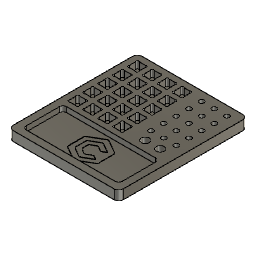
Bamboo Tray (Fusion) (Autodesk Fusion 360 design; units mm, degrees)
Autodesk Fusion 360 part; units mm, degrees
sketch "Sketch1" plane through (0, 0, 0) normal (0, 0, 1) x (1, 0, 0)
  line L0 (0, 0) -> (148, 0)
  line L1 (148, 0) -> (148, 173)
  line L2 (148, 173) -> (0, 173)
  line L3 (0, 173) -> (0, 0)
  dimension "d1" = 148
  dimension "d2" = 173
  constraint horizontal L0
  constraint vertical L1
  constraint horizontal L2
  constraint vertical L3
  constraint coincident L0.start L3.end
  measures "d1" distance of L0.start L0.end
  measures "d2" distance of L0.start L2.end
extrude "Extrude1" add sketch "Sketch1" along normal blind 12.7
sketch "Sketch2" plane through (0, 0, 12.7) normal (0, 0, 1) x (-1, 0, 0)
  line L0 (0, -173) -> (0, 0) construction
  line L1 (0, 0) -> (-148, 0) construction
  line L2 (-148, 0) -> (-148, -173) construction
  line L3 (-11.2739, -71.314) -> (-18.7691, -71.314)
  line L4 (-21.5019, -74.0964) -> (-21.5019, -81.9465)
  line L5 (-18.7712, -84.7264) -> (-11.1924, -84.7264)
  line L6 (-8.4537, -81.9513) -> (-8.4537, -74.0071)
  line L7 (-8.5338, -71.2781) -> (-21.432, -84.6864) construction
  line L8 (-21.4944, -71.3042) -> (-8.4323, -84.7713) construction
  arc A0 (-11.1924, -84.7264) -> (-8.4537, -81.9513) centre (-9.79, -83.3716) ccw
  arc A1 (-21.5019, -81.9465) -> (-18.7712, -84.7264) centre (-20.0802, -83.2811) ccw
  arc A2 (-8.4537, -74.0071) -> (-11.2739, -71.314) centre (-9.8857, -72.6834) ccw
  arc A3 (-18.7691, -71.314) -> (-21.5019, -74.0964) centre (-20.1368, -72.704) ccw
  line L9 (-28.4537, -81.9513) -> (-28.4537, -74.0071)
  arc A4 (-28.4537, -74.0071) -> (-31.2739, -71.314) centre (-29.8857, -72.6834) ccw
  line L10 (-31.2739, -71.314) -> (-38.7691, -71.314)
  arc A5 (-38.7691, -71.314) -> (-41.5019, -74.0964) centre (-40.1368, -72.704) ccw
  line L11 (-41.5019, -74.0964) -> (-41.5019, -81.9465)
  arc A6 (-41.5019, -81.9465) -> (-38.7712, -84.7264) centre (-40.0802, -83.2811) ccw
  line L12 (-38.7712, -84.7264) -> (-31.1924, -84.7264)
  arc A7 (-31.1924, -84.7264) -> (-28.4537, -81.9513) centre (-29.79, -83.3716) ccw
  line L13 (-48.4537, -81.9513) -> (-48.4537, -74.0071)
  arc A8 (-48.4537, -74.0071) -> (-51.2739, -71.314) centre (-49.8857, -72.6834) ccw
  line L14 (-51.2739, -71.314) -> (-58.7691, -71.314)
  arc A9 (-58.7691, -71.314) -> (-61.5019, -74.0964) centre (-60.1368, -72.704) ccw
  line L15 (-61.5019, -74.0964) -> (-61.5019, -81.9465)
  arc A10 (-61.5019, -81.9465) -> (-58.7712, -84.7264) centre (-60.0802, -83.2811) ccw
  line L16 (-58.7712, -84.7264) -> (-51.1924, -84.7264)
  arc A11 (-51.1924, -84.7264) -> (-48.4537, -81.9513) centre (-49.79, -83.3716) ccw
  line L17 (-68.4537, -81.9513) -> (-68.4537, -74.0071)
  arc A12 (-68.4537, -74.0071) -> (-71.2739, -71.314) centre (-69.8857, -72.6834) ccw
  line L18 (-71.2739, -71.314) -> (-78.7691, -71.314)
  arc A13 (-78.7691, -71.314) -> (-81.5019, -74.0964) centre (-80.1368, -72.704) ccw
  line L19 (-81.5019, -74.0964) -> (-81.5019, -81.9465)
  arc A14 (-81.5019, -81.9465) -> (-78.7712, -84.7264) centre (-80.0802, -83.2811) ccw
  line L20 (-78.7712, -84.7264) -> (-71.1924, -84.7264)
  arc A15 (-71.1924, -84.7264) -> (-68.4537, -81.9513) centre (-69.79, -83.3716) ccw
  line L21 (-8.4537, -101.9513) -> (-8.4537, -94.0071)
  arc A16 (-8.4537, -94.0071) -> (-11.2739, -91.314) centre (-9.8857, -92.6834) ccw
  line L22 (-11.2739, -91.314) -> (-18.7691, -91.314)
  arc A17 (-18.7691, -91.314) -> (-21.5019, -94.0964) centre (-20.1368, -92.704) ccw
  line L23 (-21.5019, -94.0964) -> (-21.5019, -101.9465)
  arc A18 (-21.5019, -101.9465) -> (-18.7712, -104.7264) centre (-20.0802, -103.2811) ccw
  line L24 (-18.7712, -104.7264) -> (-11.1924, -104.7264)
  arc A19 (-11.1924, -104.7264) -> (-8.4537, -101.9513) centre (-9.79, -103.3716) ccw
  line L25 (-28.4537, -101.9513) -> (-28.4537, -94.0071)
  arc A20 (-28.4537, -94.0071) -> (-31.2739, -91.314) centre (-29.8857, -92.6834) ccw
  line L26 (-31.2739, -91.314) -> (-38.7691, -91.314)
  arc A21 (-38.7691, -91.314) -> (-41.5019, -94.0964) centre (-40.1368, -92.704) ccw
  line L27 (-41.5019, -94.0964) -> (-41.5019, -101.9465)
  arc A22 (-41.5019, -101.9465) -> (-38.7712, -104.7264) centre (-40.0802, -103.2811) ccw
  line L28 (-38.7712, -104.7264) -> (-31.1924, -104.7264)
  arc A23 (-31.1924, -104.7264) -> (-28.4537, -101.9513) centre (-29.79, -103.3716) ccw
  line L29 (-48.4537, -101.9513) -> (-48.4537, -94.0071)
  arc A24 (-48.4537, -94.0071) -> (-51.2739, -91.314) centre (-49.8857, -92.6834) ccw
  line L30 (-51.2739, -91.314) -> (-58.7691, -91.314)
  arc A25 (-58.7691, -91.314) -> (-61.5019, -94.0964) centre (-60.1368, -92.704) ccw
  line L31 (-61.5019, -94.0964) -> (-61.5019, -101.9465)
  arc A26 (-61.5019, -101.9465) -> (-58.7712, -104.7264) centre (-60.0802, -103.2811) ccw
  line L32 (-58.7712, -104.7264) -> (-51.1924, -104.7264)
  arc A27 (-51.1924, -104.7264) -> (-48.4537, -101.9513) centre (-49.79, -103.3716) ccw
  line L33 (-68.4537, -101.9513) -> (-68.4537, -94.0071)
  arc A28 (-68.4537, -94.0071) -> (-71.2739, -91.314) centre (-69.8857, -92.6834) ccw
  line L34 (-71.2739, -91.314) -> (-78.7691, -91.314)
  arc A29 (-78.7691, -91.314) -> (-81.5019, -94.0964) centre (-80.1368, -92.704) ccw
  line L35 (-81.5019, -94.0964) -> (-81.5019, -101.9465)
  arc A30 (-81.5019, -101.9465) -> (-78.7712, -104.7264) centre (-80.0802, -103.2811) ccw
  line L36 (-78.7712, -104.7264) -> (-71.1924, -104.7264)
  arc A31 (-71.1924, -104.7264) -> (-68.4537, -101.9513) centre (-69.79, -103.3716) ccw
  line L37 (-8.4537, -121.9513) -> (-8.4537, -114.0071)
  arc A32 (-8.4537, -114.0071) -> (-11.2739, -111.314) centre (-9.8857, -112.6834) ccw
  line L38 (-11.2739, -111.314) -> (-18.7691, -111.314)
  arc A33 (-18.7691, -111.314) -> (-21.5019, -114.0964) centre (-20.1368, -112.704) ccw
  line L39 (-21.5019, -114.0964) -> (-21.5019, -121.9465)
  arc A34 (-21.5019, -121.9465) -> (-18.7712, -124.7264) centre (-20.0802, -123.2811) ccw
  line L40 (-18.7712, -124.7264) -> (-11.1924, -124.7264)
  arc A35 (-11.1924, -124.7264) -> (-8.4537, -121.9513) centre (-9.79, -123.3716) ccw
  line L41 (-28.4537, -121.9513) -> (-28.4537, -114.0071)
  arc A36 (-28.4537, -114.0071) -> (-31.2739, -111.314) centre (-29.8857, -112.6834) ccw
  line L42 (-31.2739, -111.314) -> (-38.7691, -111.314)
  arc A37 (-38.7691, -111.314) -> (-41.5019, -114.0964) centre (-40.1368, -112.704) ccw
  line L43 (-41.5019, -114.0964) -> (-41.5019, -121.9465)
  arc A38 (-41.5019, -121.9465) -> (-38.7712, -124.7264) centre (-40.0802, -123.2811) ccw
  line L44 (-38.7712, -124.7264) -> (-31.1924, -124.7264)
  arc A39 (-31.1924, -124.7264) -> (-28.4537, -121.9513) centre (-29.79, -123.3716) ccw
  line L45 (-48.4537, -121.9513) -> (-48.4537, -114.0071)
  arc A40 (-48.4537, -114.0071) -> (-51.2739, -111.314) centre (-49.8857, -112.6834) ccw
  line L46 (-51.2739, -111.314) -> (-58.7691, -111.314)
  arc A41 (-58.7691, -111.314) -> (-61.5019, -114.0964) centre (-60.1368, -112.704) ccw
  line L47 (-61.5019, -114.0964) -> (-61.5019, -121.9465)
  arc A42 (-61.5019, -121.9465) -> (-58.7712, -124.7264) centre (-60.0802, -123.2811) ccw
  line L48 (-58.7712, -124.7264) -> (-51.1924, -124.7264)
  arc A43 (-51.1924, -124.7264) -> (-48.4537, -121.9513) centre (-49.79, -123.3716) ccw
  line L49 (-68.4537, -121.9513) -> (-68.4537, -114.0071)
  arc A44 (-68.4537, -114.0071) -> (-71.2739, -111.314) centre (-69.8857, -112.6834) ccw
  line L50 (-71.2739, -111.314) -> (-78.7691, -111.314)
  arc A45 (-78.7691, -111.314) -> (-81.5019, -114.0964) centre (-80.1368, -112.704) ccw
  line L51 (-81.5019, -114.0964) -> (-81.5019, -121.9465)
  arc A46 (-81.5019, -121.9465) -> (-78.7712, -124.7264) centre (-80.0802, -123.2811) ccw
  line L52 (-78.7712, -124.7264) -> (-71.1924, -124.7264)
  arc A47 (-71.1924, -124.7264) -> (-68.4537, -121.9513) centre (-69.79, -123.3716) ccw
  line L53 (-8.4537, -141.9513) -> (-8.4537, -134.0071)
  arc A48 (-8.4537, -134.0071) -> (-11.2739, -131.314) centre (-9.8857, -132.6834) ccw
  line L54 (-11.2739, -131.314) -> (-18.7691, -131.314)
  arc A49 (-18.7691, -131.314) -> (-21.5019, -134.0964) centre (-20.1368, -132.704) ccw
  line L55 (-21.5019, -134.0964) -> (-21.5019, -141.9465)
  arc A50 (-21.5019, -141.9465) -> (-18.7712, -144.7264) centre (-20.0802, -143.2811) ccw
  line L56 (-18.7712, -144.7264) -> (-11.1924, -144.7264)
  arc A51 (-11.1924, -144.7264) -> (-8.4537, -141.9513) centre (-9.79, -143.3716) ccw
  line L57 (-28.4537, -141.9513) -> (-28.4537, -134.0071)
  arc A52 (-28.4537, -134.0071) -> (-31.2739, -131.314) centre (-29.8857, -132.6834) ccw
  line L58 (-31.2739, -131.314) -> (-38.7691, -131.314)
  arc A53 (-38.7691, -131.314) -> (-41.5019, -134.0964) centre (-40.1368, -132.704) ccw
  line L59 (-41.5019, -134.0964) -> (-41.5019, -141.9465)
  arc A54 (-41.5019, -141.9465) -> (-38.7712, -144.7264) centre (-40.0802, -143.2811) ccw
  line L60 (-38.7712, -144.7264) -> (-31.1924, -144.7264)
  arc A55 (-31.1924, -144.7264) -> (-28.4537, -141.9513) centre (-29.79, -143.3716) ccw
  line L61 (-48.4537, -141.9513) -> (-48.4537, -134.0071)
  arc A56 (-48.4537, -134.0071) -> (-51.2739, -131.314) centre (-49.8857, -132.6834) ccw
  line L62 (-51.2739, -131.314) -> (-58.7691, -131.314)
  arc A57 (-58.7691, -131.314) -> (-61.5019, -134.0964) centre (-60.1368, -132.704) ccw
  line L63 (-61.5019, -134.0964) -> (-61.5019, -141.9465)
  arc A58 (-61.5019, -141.9465) -> (-58.7712, -144.7264) centre (-60.0802, -143.2811) ccw
  line L64 (-58.7712, -144.7264) -> (-51.1924, -144.7264)
  arc A59 (-51.1924, -144.7264) -> (-48.4537, -141.9513) centre (-49.79, -143.3716) ccw
  line L65 (-68.4537, -141.9513) -> (-68.4537, -134.0071)
  arc A60 (-68.4537, -134.0071) -> (-71.2739, -131.314) centre (-69.8857, -132.6834) ccw
  line L66 (-71.2739, -131.314) -> (-78.7691, -131.314)
  arc A61 (-78.7691, -131.314) -> (-81.5019, -134.0964) centre (-80.1368, -132.704) ccw
  line L67 (-81.5019, -134.0964) -> (-81.5019, -141.9465)
  arc A62 (-81.5019, -141.9465) -> (-78.7712, -144.7264) centre (-80.0802, -143.2811) ccw
  line L68 (-78.7712, -144.7264) -> (-71.1924, -144.7264)
  arc A63 (-71.1924, -144.7264) -> (-68.4537, -141.9513) centre (-69.79, -143.3716) ccw
  line L69 (-8.4537, -161.9513) -> (-8.4537, -154.0071)
  arc A64 (-8.4537, -154.0071) -> (-11.2739, -151.314) centre (-9.8857, -152.6834) ccw
  line L70 (-11.2739, -151.314) -> (-18.7691, -151.314)
  arc A65 (-18.7691, -151.314) -> (-21.5019, -154.0964) centre (-20.1368, -152.704) ccw
  line L71 (-21.5019, -154.0964) -> (-21.5019, -161.9465)
  arc A66 (-21.5019, -161.9465) -> (-18.7712, -164.7264) centre (-20.0802, -163.2811) ccw
  line L72 (-18.7712, -164.7264) -> (-11.1924, -164.7264)
  arc A67 (-11.1924, -164.7264) -> (-8.4537, -161.9513) centre (-9.79, -163.3716) ccw
  line L73 (-28.4537, -161.9513) -> (-28.4537, -154.0071)
  arc A68 (-28.4537, -154.0071) -> (-31.2739, -151.314) centre (-29.8857, -152.6834) ccw
  line L74 (-31.2739, -151.314) -> (-38.7691, -151.314)
  arc A69 (-38.7691, -151.314) -> (-41.5019, -154.0964) centre (-40.1368, -152.704) ccw
  line L75 (-41.5019, -154.0964) -> (-41.5019, -161.9465)
  arc A70 (-41.5019, -161.9465) -> (-38.7712, -164.7264) centre (-40.0802, -163.2811) ccw
  line L76 (-38.7712, -164.7264) -> (-31.1924, -164.7264)
  arc A71 (-31.1924, -164.7264) -> (-28.4537, -161.9513) centre (-29.79, -163.3716) ccw
  line L77 (-48.4537, -161.9513) -> (-48.4537, -154.0071)
  arc A72 (-48.4537, -154.0071) -> (-51.2739, -151.314) centre (-49.8857, -152.6834) ccw
  line L78 (-51.2739, -151.314) -> (-58.7691, -151.314)
  arc A73 (-58.7691, -151.314) -> (-61.5019, -154.0964) centre (-60.1368, -152.704) ccw
  line L79 (-61.5019, -154.0964) -> (-61.5019, -161.9465)
  arc A74 (-61.5019, -161.9465) -> (-58.7712, -164.7264) centre (-60.0802, -163.2811) ccw
  line L80 (-58.7712, -164.7264) -> (-51.1924, -164.7264)
  arc A75 (-51.1924, -164.7264) -> (-48.4537, -161.9513) centre (-49.79, -163.3716) ccw
  line L81 (-68.4537, -161.9513) -> (-68.4537, -154.0071)
  arc A76 (-68.4537, -154.0071) -> (-71.2739, -151.314) centre (-69.8857, -152.6834) ccw
  line L82 (-71.2739, -151.314) -> (-78.7691, -151.314)
  arc A77 (-78.7691, -151.314) -> (-81.5019, -154.0964) centre (-80.1368, -152.704) ccw
  line L83 (-81.5019, -154.0964) -> (-81.5019, -161.9465)
  arc A78 (-81.5019, -161.9465) -> (-78.7712, -164.7264) centre (-80.0802, -163.2811) ccw
  line L84 (-78.7712, -164.7264) -> (-71.1924, -164.7264)
  arc A79 (-71.1924, -164.7264) -> (-68.4537, -161.9513) centre (-69.79, -163.3716) ccw
  line L85 (-148, -173) -> (0, -173)
  circle A80 centre (-133, -160.5) radius 3.275
  circle A81 centre (-116, -160.5) radius 3.275
  circle A82 centre (-99, -160.5) radius 3.275
  circle A83 centre (-133, -143.5) radius 3.275
  circle A84 centre (-116, -143.5) radius 3.275
  circle A85 centre (-99, -143.5) radius 3.275
  circle A86 centre (-133, -126.5) radius 3.275
  circle A87 centre (-116, -126.5) radius 3.275
  circle A88 centre (-99, -126.5) radius 3.275
  circle A89 centre (-133, -109.5) radius 3.275
  circle A90 centre (-116, -109.5) radius 3.275
  circle A91 centre (-99, -109.5) radius 3.275
  circle A92 centre (-133, -92.5) radius 3.275
  circle A93 centre (-116, -92.5) radius 3.275
  circle A94 centre (-99, -92.5) radius 3.275
  line L86 (-99, -92.5) -> (-116, -92.5) construction
  circle A95 centre (-106.2904, -77.5) radius 5.375
  circle A96 centre (-126.2904, -77.5) radius 5.375
  line L87 (-138.5, -9.5) -> (-9.5, -9.5)
  line L88 (-9.5, -9.5) -> (-9.5, -63.814)
  line L89 (-9.5, -63.814) -> (-138.5, -63.814)
  line L90 (-138.5, -63.814) -> (-138.5, -9.5)
  line L91 (-138.5, -9.5) -> (-9.5, -63.814) construction
  line L92 (-9.5, -9.5) -> (-138.5, -63.814) construction
  line L93 (-106.2904, -92.5) -> (-106.2904, -77.5) construction
  line L94 (-126.2904, -77.5) -> (-106.2904, -77.5) construction
  point P0 (-15, -78)
  point P1 (-106.2904, -92.5)
  point P2 (-81.5019, -78.0214)
  point P3 (-74, -36.657)
  dimension "d6" = 13
  dimension "d8" = 15
  dimension "d13" = 3.9
  dimension "d14" = 3.9
  dimension "d15" = 3.9
  dimension "d16" = 3.9
  dimension "d19" = -20
  dimension "d20" = -20
  dimension "d27" = 95
  dimension "d28" = 6.55
  dimension "d30" = 30
  dimension "d31" = 50
  dimension "d32" = 17
  dimension "d33" = 17
  dimension "d34" = 15
  dimension "d35" = 12.5
  dimension "d49" = 9.5
  dimension "d50" = 9.5
  dimension "d51" = 9.5
  dimension "d52" = 7.5
  dimension "d56" = 15
  dimension "d61" = 10.75
  dimension "d62" = 20
  dimension "d63" = 9.7096
  constraint perpendicular L3 L4
  constraint parallel L3 L5
  constraint parallel L4 L6
  constraint horizontal L3
  constraint coincident L7 P0
  constraint coincident L8 P0
  constraint coincident L8 A0.centre
  constraint coincident L8.end A0
  constraint coincident L7 A1.centre
  constraint coincident L7.end A1
  constraint coincident L8 A3.centre
  constraint coincident L8.start A3
  constraint coincident L7 A2.centre
  constraint coincident L7.start A2
  constraint coincident A94.centre L86.start
  constraint coincident A93.centre L86.end
  constraint midpoint L19 P2
  constraint horizontal L87
  constraint perpendicular L87 L88
  constraint parallel L87 L89
  constraint parallel L88 L90
  constraint coincident L91 P3
  constraint coincident L92 P3
  constraint coincident P1 L93.start
  constraint coincident A95.centre L93.end
  constraint vertical L93
  constraint equal A95 A96
  constraint coincident A96.centre L94.start
  constraint perpendicular L93 L94
  measures "d6" distance of L7.end L8.end
  measures "d8" distance of L0 P0
  measures "d13" diameter of A0
  measures "d14" diameter of A1
  measures "d15" diameter of A3
  measures "d16" diameter of A2
  measures "d27" distance of P0 L85
  measures "d28" diameter of A80
  measures "d34" distance of L2 A80.centre
  measures "d35" distance of L85 A80.centre
  measures "d49" distance of L1 L87
  measures "d50" distance of L2 L90
  measures "d51" distance of L0 L88
  measures "d52" distance of L3 L89
  measures "d56" distance of P1 A95.centre
  measures "d61" diameter of A96
  measures "d62" distance of A95.centre A96.centre
  measures "d63" distance of A93.centre A95.centre
extrude "Extrude2" cut sketch "Sketch2" against normal blind 9.5 contours L3 L4 L5 L6 A0 A1 A2 A3 | L9 A4 L10 A5 L11 A6 L12 A7 | L13 A8 L14 A9 L15 A10 L16 A11 | L17 A12 L18 A13 L19 A14 L20 A15 | L21 A16 L22 A17 L23 A18 L24 A19 | L25 A20 L26 A21 L27 A22 L28 A23 | L29 A24 L30 A25 L31 A26 L32 A27 | L33 A28 L34 A29 L35 A30 L36 A31 | L37 A32 L38 A33 L39 A34 L40 A35 | L41 A36 L42 A37 L43 A38 L44 A39 | L45 A40 L46 A41 L47 A42 L48 A43 | L49 A44 L50 A45 L51 A46 L52 A47 | L53 A48 L54 A49 L55 A50 L56 A51 | L57 A52 L58 A53 L59 A54 L60 A55 | L61 A56 L62 A57 L63 A58 L64 A59 | L65 A60 L66 A61 L67 A62 L68 A63 | L69 A64 L70 A65 L71 A66 L72 A67 | L73 A68 L74 A69 L75 A70 L76 A71 | L77 A72 L78 A73 L79 A74 L80 A75 | L81 A76 L82 A77 L83 A78 L84 A79 | A80 | A81 | A82 | A83 | A84 | A85 | A86 | A87 | A88 | A89 | A90 | A91 | A92 | A93 | A94
fillet "Fillet1" radius 6 4 edges at (0, 0, 6.35) (148, 0, 6.35) (148, 173, 6.35) (0, 173, 6.35)
ref_plane "WorkPlane1" through (104.5, 75, 7.45) normal (0, 1, 0) x (0, 0, -1)
sketch "Sketch3" plane through (104.5, 75, 7.45) normal (0, 1, 0) x (1, 0, 0)
  line L0 (4.6, -5.25) -> (-4.6, -5.25)
  line L1 (4.6, 5.25) -> (-4.6, 5.25)
  line L2 (4.6, -5.25) -> (-4.6, -5.25)
  line L3 (0, 0) -> (0, -5.25)
  line L4 (4.6, -5.25) -> (3.1243, 5.25) construction
  line L5 (4.6, -5.25) -> (15.1032, -5.25) construction
  line L6 (4.6, 5.25) -> (4.6, 1.25)
  line L7 (4.6, 1.25) -> (3.6865, 1.25)
  line L8 (3.6865, 1.25) -> (3.6865, 5.25)
  line L9 (3.6865, 5.25) -> (4.6, 5.25)
  dimension "d40" = 98
  dimension "d41" = 4
  constraint coincident L3.start origin
  constraint midpoint L0 L3.end
  constraint horizontal L5
  constraint coincident L0.start L2.start
  constraint coincident L1 L4.end
  constraint coincident L1.start L6.start
  constraint perpendicular L1 L6
  constraint coincident L4 L7.end
  constraint perpendicular L6 L7
  constraint coincident L1 L8.end
  constraint perpendicular L1 L8
  measures "d40" angle of L4 L5
  measures "d41" distance of L1.start L6.end
revolve "Revolve1" [suppressed]
extrude "Extrude3" cut sketch "Sketch2" against normal blind 10.5 draft -8 contours A95 | A96
extrude "Extrude4" cut sketch "Sketch2" against normal blind 7 contours L87 L88 L89 L90
fillet "Fillet2" radius 5 4 edges at (9.5, 63.814, 9.2) (9.5, 9.5, 9.2) (138.5, 63.814, 9.2) (138.5, 9.5, 9.2)
sketch "Sketch4" plane through (0, 0, 5.7) normal (0, 0, 1) x (-1, 0, 0)
  arc A0 (-133.5, -9.5) -> (-138.5, -14.5) centre (-133.5, -14.5) ccw
  line L0 (-138.5, -14.5) -> (-138.5, -58.814)
  arc A1 (-138.5, -58.814) -> (-133.5, -63.814) centre (-133.5, -58.814) ccw
  line L1 (-133.5, -63.814) -> (-14.5, -63.814)
  arc A2 (-14.5, -63.814) -> (-9.5, -58.814) centre (-14.5, -58.814) ccw
  line L2 (-9.5, -58.814) -> (-9.5, -14.5)
  arc A3 (-9.5, -14.5) -> (-14.5, -9.5) centre (-14.5, -14.5) ccw
  line L3 (-14.5, -9.5) -> (-133.5, -9.5)
  line L4 (-75.1019, -28.3976) -> (-80.9582, -31.7787)
  arc A4 (-72.8981, -28.3976) -> (-75.1019, -28.3976) centre (-74, -30.3062) ccw
  arc A5 (-65.9399, -33.6873) -> (-67.0418, -31.7787) centre (-68.1438, -33.6873) ccw
  line L5 (-65.9399, -40.4495) -> (-65.9399, -33.6873)
  line L6 (-72.8981, -45.7392) -> (-67.0418, -42.3581)
  arc A6 (-67.0418, -42.3581) -> (-65.9399, -40.4495) centre (-68.1438, -40.4495) ccw
  line L7 (-67.0418, -31.7787) -> (-72.8981, -28.3976)
  arc A7 (-60.0441, -43.8607) -> (-61.0054, -45.6809) centre (-62.248, -43.8607) cw
  line L8 (-60.0441, -30.2834) -> (-60.0441, -43.8607)
  arc A8 (-61.146, -28.3747) -> (-60.0441, -30.2834) centre (-62.248, -30.2834) cw
  arc A9 (-72.8981, -52.5471) -> (-75.1019, -52.5471) centre (-74, -50.6385) cw
  line L9 (-87.1295, -44.6487) -> (-83.1621, -42.3581)
  line L10 (-75.1019, -52.5471) -> (-87.1295, -45.603)
  arc A10 (-87.1295, -29.4881) -> (-87.1295, -28.5338) centre (-86.854, -29.0109) cw
  arc A11 (-75.1019, -21.5897) -> (-72.8981, -21.5897) centre (-74, -23.4983) cw
  line L11 (-72.8981, -21.5897) -> (-61.146, -28.3747)
  line L12 (-87.1295, -28.5338) -> (-75.1019, -21.5897)
  arc A12 (-83.1621, -42.3581) -> (-80.9582, -42.3581) centre (-82.0601, -44.2667) cw
  arc A13 (-87.1295, -45.603) -> (-87.1295, -44.6487) centre (-86.854, -45.1259) cw
  line L13 (-61.0054, -45.6809) -> (-72.8981, -52.5471)
  line L14 (-80.9582, -42.3581) -> (-75.1019, -45.7392)
  arc A14 (-75.1019, -45.7392) -> (-72.8981, -45.7392) centre (-74, -43.8306) ccw
  line L15 (-83.1621, -31.7787) -> (-87.1295, -29.4881)
  arc A15 (-80.9582, -31.7787) -> (-83.1621, -31.7787) centre (-82.0601, -29.87) cw
  line L16 (-74, -63.814) -> (-74, -9.5) construction
  arc A16 (-94.2793, -26.6328) -> (-93.1774, -24.7242) centre (-92.0754, -26.6328) cw
  arc A17 (-54.8229, -24.7238) -> (-53.7209, -26.6324) centre (-55.9248, -26.6324) cw
  line L17 (-93.1774, -24.7242) -> (-75.1022, -14.2882)
  arc A18 (-53.7207, -47.504) -> (-54.8226, -49.4126) centre (-55.9246, -47.504) cw
  line L18 (-53.7209, -26.6324) -> (-53.7207, -47.504)
  line L19 (-54.8226, -49.4126) -> (-72.8978, -59.8486)
  line L20 (-94.2791, -47.5044) -> (-94.2793, -26.6328)
  arc A19 (-93.1771, -49.413) -> (-94.2791, -47.5044) centre (-92.0752, -47.5044) cw
  arc A20 (-75.1022, -14.2882) -> (-72.8983, -14.2882) centre (-74.0002, -16.1968) cw
  arc A21 (-72.8978, -59.8486) -> (-75.1017, -59.8486) centre (-73.9998, -57.94) cw
  line L21 (-75.1017, -59.8486) -> (-93.1771, -49.413)
  line L22 (-72.8983, -14.2882) -> (-54.8229, -24.7238)
  point P0 (-74, -36.657)
  constraint midpoint L1 L16.start
  constraint midpoint L3 L16.end
  constraint midpoint L16 P0
sketch "Sketch5" plane through (0, 0, 4.7) normal (0, 0, 1) x (-1, 0, 0)
  arc A0 (-133, -10) -> (-138, -15) centre (-133, -15) ccw
  line L0 (-138, -15) -> (-138, -58.814)
  arc A1 (-138, -58.814) -> (-133, -63.814) centre (-133, -58.814) ccw
  line L1 (-133, -63.814) -> (-15, -63.814)
  arc A2 (-15, -63.814) -> (-10, -58.814) centre (-15, -58.814) ccw
  line L2 (-10, -58.814) -> (-10, -15)
  arc A3 (-10, -15) -> (-15, -10) centre (-15, -15) ccw
  line L3 (-15, -10) -> (-133, -10)
  line L4 (-74, -63.814) -> (-74, -10) construction
  line L5 (-138, -36.907) -> (-10, -36.907) construction
  line L6 (-44.0656, -28.0911) -> (-44.0656, -45.4544)
  line L7 (-44.0656, -45.4544) -> (-42.6997, -45.4544)
  line L8 (-42.6997, -45.4544) -> (-42.7229, -32.6519)
  line L9 (-42.7229, -32.6519) -> (-42.7692, -30.7998)
  line L10 (-42.7692, -30.7998) -> (-42.7229, -30.7766)
  line L11 (-42.7229, -30.7766) -> (-41.7042, -32.3509)
  line L12 (-41.7042, -32.3509) -> (-33.0226, -45.4544)
  line L13 (-33.0226, -45.4544) -> (-31.5178, -45.4544)
  line L14 (-31.5178, -45.4544) -> (-31.5178, -28.0911)
  line L15 (-31.5178, -28.0911) -> (-32.9069, -28.0911)
  line L16 (-32.9069, -28.0911) -> (-32.9069, -41.1946)
  line L17 (-32.9069, -41.1946) -> (-32.8837, -43.0698)
  line L18 (-32.8837, -43.0698) -> (-32.93, -43.093)
  line L19 (-32.93, -43.093) -> (-33.9486, -41.5187)
  line L20 (-33.9486, -41.5187) -> (-42.9312, -28.0911)
  line L21 (-42.9312, -28.0911) -> (-44.0656, -28.0911)
  spline S0 degree 3 poles (-62.1003, -36.7728) (-62.1003, -43.2087) (-60.2251, -45.7322) (-55.1781, -45.7322) knots 0 0 0 0 1 1 1 1
  spline S1 degree 3 poles (-55.1781, -45.7322) (-50.1544, -45.7322) (-48.256, -43.2087) (-48.256, -36.7728) knots 0 0 0 0 1 1 1 1
  spline S2 degree 3 poles (-48.256, -36.7728) (-48.256, -30.3368) (-50.1775, -27.767) (-55.1781, -27.767) knots 0 0 0 0 1 1 1 1
  spline S3 degree 3 poles (-55.1781, -27.767) (-60.2251, -27.767) (-62.1003, -30.3136) (-62.1003, -36.7728) knots 0 0 0 0 1 1 1 1
  spline S4 degree 3 poles (-60.526, -36.7728) (-60.526, -30.9387) (-59.0212, -29.2487) (-55.2013, -29.2487) knots 0 0 0 0 1 1 1 1
  spline S5 degree 3 poles (-55.2013, -29.2487) (-51.3582, -29.2487) (-49.8302, -30.9387) (-49.8302, -36.7728) knots 0 0 0 0 1 1 1 1
  spline S6 degree 3 poles (-49.8302, -36.7728) (-49.8302, -42.63) (-51.3582, -44.2737) (-55.1781, -44.2737) knots 0 0 0 0 1 1 1 1
  spline S7 degree 3 poles (-55.1781, -44.2737) (-59.0212, -44.2737) (-60.526, -42.63) (-60.526, -36.7728) knots 0 0 0 0 1 1 1 1
  line L22 (-66.2676, -45.4544) -> (-66.2676, -28.0911)
  line L23 (-66.2676, -28.0911) -> (-67.6103, -28.0911)
  line L24 (-67.6103, -28.0911) -> (-67.6103, -41.0094)
  line L25 (-67.6103, -41.0094) -> (-67.5872, -42.8846)
  line L26 (-67.5872, -42.8846) -> (-67.6335, -42.9078)
  line L27 (-67.6335, -42.9078) -> (-68.3048, -41.1483)
  line L28 (-68.3048, -41.1483) -> (-73.6527, -28.0911)
  line L29 (-73.6527, -28.0911) -> (-74.8103, -28.0911)
  line L30 (-74.8103, -28.0911) -> (-80.1582, -41.2177)
  line L31 (-80.1582, -41.2177) -> (-80.8295, -42.9772)
  line L32 (-80.8295, -42.9772) -> (-80.899, -42.9541)
  line L33 (-80.899, -42.9541) -> (-80.8527, -41.0788)
  line L34 (-80.8527, -41.0788) -> (-80.8527, -28.0911)
  line L35 (-80.8527, -28.0911) -> (-82.2186, -28.0911)
  line L36 (-82.2186, -28.0911) -> (-82.2186, -45.4544)
  line L37 (-82.2186, -45.4544) -> (-80.436, -45.4544)
  line L38 (-80.436, -45.4544) -> (-74.9492, -31.9573)
  line L39 (-74.9492, -31.9573) -> (-74.301, -30.221)
  line L40 (-74.301, -30.221) -> (-74.2315, -30.221)
  line L41 (-74.2315, -30.221) -> (-73.5601, -31.9573)
  line L42 (-73.5601, -31.9573) -> (-68.0733, -45.4544)
  line L43 (-68.0733, -45.4544) -> (-66.2676, -45.4544)
  line L44 (-98.6559, -28.0911) -> (-100.369, -28.0911)
  line L45 (-100.369, -28.0911) -> (-93.771, -45.4544)
  line L46 (-93.771, -45.4544) -> (-91.9652, -45.4544)
  line L47 (-91.9652, -45.4544) -> (-85.3672, -28.0911)
  line L48 (-85.3672, -28.0911) -> (-87.0109, -28.0911)
  line L49 (-87.0109, -28.0911) -> (-88.6546, -32.675)
  line L50 (-88.6546, -32.675) -> (-97.0121, -32.675)
  line L51 (-97.0121, -32.675) -> (-98.6559, -28.0911)
  line L52 (-92.8449, -44.32) -> (-92.9144, -44.32)
  line L53 (-92.9144, -44.32) -> (-93.4932, -42.5374)
  line L54 (-93.4932, -42.5374) -> (-96.526, -34.0409)
  line L55 (-96.526, -34.0409) -> (-89.1639, -34.0409)
  line L56 (-89.1639, -34.0409) -> (-92.243, -42.5374)
  line L57 (-92.243, -42.5374) -> (-92.8449, -44.32)
  spline S8 degree 3 poles (-116.4821, -36.8422) (-116.4821, -43.0004) (-114.306, -45.4544) (-109.1896, -45.4544) knots 0 0 0 0 1 1 1 1
  line L58 (-109.1896, -45.4544) -> (-103.5176, -45.4544)
  line L59 (-103.5176, -45.4544) -> (-103.5176, -28.0911)
  line L60 (-103.5176, -28.0911) -> (-109.2127, -28.0911)
  spline S9 degree 3 poles (-109.2127, -28.0911) (-114.1439, -28.0911) (-116.4821, -30.4988) (-116.4821, -36.8422) knots 0 0 0 0 1 1 1 1
  spline S10 degree 3 poles (-114.8847, -36.8422) (-114.8847, -31.1008) (-112.9863, -29.5496) (-109.1664, -29.5496) knots 0 0 0 0 1 1 1 1
  line L61 (-109.1664, -29.5496) -> (-105.0455, -29.5496)
  line L62 (-105.0455, -29.5496) -> (-105.0455, -43.9727)
  line L63 (-105.0455, -43.9727) -> (-109.1433, -43.9727)
  spline S11 degree 3 poles (-109.1433, -43.9727) (-113.1716, -43.9727) (-114.8847, -42.329) (-114.8847, -36.8422) knots 0 0 0 0 1 1 1 1
  spline S12 degree 3 poles (-127.5586, -43.3862) (-127.5586, -45.0068) (-126.6634, -45.8402) (-125.0428, -46.1644) knots 0 0 0 0 1 1 1 1
  line L64 (-125.0428, -46.1644) -> (-125.0428, -46.1952)
  spline S13 degree 3 poles (-125.0428, -46.1952) (-126.293, -46.5348) (-127.219, -47.3219) (-127.219, -48.8344) knots 0 0 0 0 1 1 1 1
  spline S14 degree 3 poles (-127.219, -48.8344) (-127.219, -50.6711) (-125.8454, -51.6434) (-123.592, -51.6434) knots 0 0 0 0 1 1 1 1
  spline S15 degree 3 poles (-123.592, -51.6434) (-122.1104, -51.6434) (-120.8911, -51.0569) (-120.1194, -50.347) knots 0 0 0 0 1 1 1 1
  line L65 (-120.1194, -50.347) -> (-120.4126, -49.5598)
  spline S16 degree 3 poles (-120.4126, -49.5598) (-121.2769, -50.2852) (-122.2493, -50.7328) (-123.5457, -50.7328) knots 0 0 0 0 1 1 1 1
  spline S17 degree 3 poles (-123.5457, -50.7328) (-125.228, -50.7328) (-126.3084, -50.1155) (-126.3084, -48.7727) knots 0 0 0 0 1 1 1 1
  spline S18 degree 3 poles (-126.3084, -48.7727) (-126.3084, -47.3373) (-125.2589, -46.5348) (-122.5888, -46.5348) knots 0 0 0 0 1 1 1 1
  line L66 (-122.5888, -46.5348) -> (-122.5888, -45.7631)
  spline S19 degree 3 poles (-122.5888, -45.7631) (-125.475, -45.7631) (-126.6171, -45.084) (-126.6171, -43.448) knots 0 0 0 0 1 1 1 1
  spline S20 degree 3 poles (-126.6171, -43.448) (-126.6171, -41.8583) (-125.6293, -40.7007) (-123.4531, -40.7007) knots 0 0 0 0 1 1 1 1
  spline S21 degree 3 poles (-123.4531, -40.7007) (-122.1412, -40.7007) (-121.138, -41.0248) (-120.2428, -41.6113) knots 0 0 0 0 1 1 1 1
  line L67 (-120.2428, -41.6113) -> (-120.0113, -40.7625)
  spline S22 degree 3 poles (-120.0113, -40.7625) (-120.8139, -40.2531) (-121.8788, -39.821) (-123.4685, -39.821) knots 0 0 0 0 1 1 1 1
  spline S23 degree 3 poles (-123.4685, -39.821) (-126.293, -39.821) (-127.5586, -41.2563) (-127.5586, -43.3862) knots 0 0 0 0 1 1 1 1
  constraint midpoint L1 L4.start
  constraint midpoint L3 L4.end
  constraint midpoint L0 L5.start
  constraint midpoint L2 L5.end
extrude "Extrude5" cut sketch "Sketch4" against normal blind 0.5 contours A16 A17 L17 A18 L18 L19 L20 A19 A20 A21 L21 L22
sketch "2D Projection" plane through (0, 0, 12.7) normal (0, 0, 1) x (-1, 0, 0)
  line L0 (-9.5, -14.5) -> (-9.5, -58.814)
  arc A0 (-14.5, -63.814) -> (-9.5, -58.814) centre (-14.5, -58.814) ccw
  line L1 (-14.5, -63.814) -> (-133.5, -63.814)
  arc A1 (-138.5, -58.814) -> (-133.5, -63.814) centre (-133.5, -58.814) ccw
  line L2 (-138.5, -58.814) -> (-138.5, -14.5)
  arc A2 (-133.5, -9.5) -> (-138.5, -14.5) centre (-133.5, -14.5) ccw
  line L3 (-133.5, -9.5) -> (-14.5, -9.5)
  arc A3 (-9.5, -14.5) -> (-14.5, -9.5) centre (-14.5, -14.5) ccw
  circle A4 centre (-106.2904, -77.5) radius 5.375
  circle A5 centre (-126.2904, -77.5) radius 5.375
  arc A6 (-6, -173) -> (0, -167) centre (-6, -167) ccw
  line L4 (0, -167) -> (0, -6)
  arc A7 (0, -6) -> (-6, 0) centre (-6, -6) ccw
  line L5 (-6, 0) -> (-142, 0)
  arc A8 (-142, 0) -> (-148, -6) centre (-142, -6) ccw
  line L6 (-148, -6) -> (-148, -167)
  arc A9 (-148, -167) -> (-142, -173) centre (-142, -167) ccw
  line L7 (-142, -173) -> (-6, -173)
  line L8 (-28.4537, -74.0071) -> (-28.4537, -81.9513)
  arc A10 (-31.1924, -84.7264) -> (-28.4537, -81.9513) centre (-29.79, -83.3716) ccw
  line L9 (-31.1924, -84.7264) -> (-38.7712, -84.7264)
  arc A11 (-41.5019, -81.9465) -> (-38.7712, -84.7264) centre (-40.0802, -83.2811) ccw
  line L10 (-41.5019, -81.9465) -> (-41.5019, -74.0964)
  arc A12 (-38.7691, -71.314) -> (-41.5019, -74.0964) centre (-40.1368, -72.704) ccw
  line L11 (-38.7691, -71.314) -> (-31.2739, -71.314)
  arc A13 (-28.4537, -74.0071) -> (-31.2739, -71.314) centre (-29.8857, -72.6834) ccw
  circle A14 centre (-133, -92.5) radius 3.275
  line L12 (-8.4537, -94.0071) -> (-8.4537, -101.9513)
  arc A15 (-11.1924, -104.7264) -> (-8.4537, -101.9513) centre (-9.79, -103.3716) ccw
  line L13 (-11.1924, -104.7264) -> (-18.7712, -104.7264)
  arc A16 (-21.5019, -101.9465) -> (-18.7712, -104.7264) centre (-20.0802, -103.2811) ccw
  line L14 (-21.5019, -101.9465) -> (-21.5019, -94.0964)
  arc A17 (-18.7691, -91.314) -> (-21.5019, -94.0964) centre (-20.1368, -92.704) ccw
  line L15 (-18.7691, -91.314) -> (-11.2739, -91.314)
  arc A18 (-8.4537, -94.0071) -> (-11.2739, -91.314) centre (-9.8857, -92.6834) ccw
  circle A19 centre (-99, -109.5) radius 3.275
  circle A20 centre (-116, -160.5) radius 3.275
  line L16 (-48.4537, -134.0071) -> (-48.4537, -141.9513)
  arc A21 (-51.1924, -144.7264) -> (-48.4537, -141.9513) centre (-49.79, -143.3716) ccw
  line L17 (-51.1924, -144.7264) -> (-58.7712, -144.7264)
  arc A22 (-61.5019, -141.9465) -> (-58.7712, -144.7264) centre (-60.0802, -143.2811) ccw
  line L18 (-61.5019, -141.9465) -> (-61.5019, -134.0964)
  arc A23 (-58.7691, -131.314) -> (-61.5019, -134.0964) centre (-60.1368, -132.704) ccw
  line L19 (-58.7691, -131.314) -> (-51.2739, -131.314)
  arc A24 (-48.4537, -134.0071) -> (-51.2739, -131.314) centre (-49.8857, -132.6834) ccw
  circle A25 centre (-116, -126.5) radius 3.275
  circle A26 centre (-99, -143.5) radius 3.275
  line L20 (-21.5019, -81.9465) -> (-21.5019, -74.0964)
  arc A27 (-18.7691, -71.314) -> (-21.5019, -74.0964) centre (-20.1368, -72.704) ccw
  line L21 (-18.7691, -71.314) -> (-11.2739, -71.314)
  arc A28 (-8.4537, -74.0071) -> (-11.2739, -71.314) centre (-9.8857, -72.6834) ccw
  line L22 (-8.4537, -74.0071) -> (-8.4537, -81.9513)
  arc A29 (-11.1924, -84.7264) -> (-8.4537, -81.9513) centre (-9.79, -83.3716) ccw
  line L23 (-11.1924, -84.7264) -> (-18.7712, -84.7264)
  arc A30 (-21.5019, -81.9465) -> (-18.7712, -84.7264) centre (-20.0802, -83.2811) ccw
  line L24 (-28.4537, -134.0071) -> (-28.4537, -141.9513)
  arc A31 (-31.1924, -144.7264) -> (-28.4537, -141.9513) centre (-29.79, -143.3716) ccw
  line L25 (-31.1924, -144.7264) -> (-38.7712, -144.7264)
  arc A32 (-41.5019, -141.9465) -> (-38.7712, -144.7264) centre (-40.0802, -143.2811) ccw
  line L26 (-41.5019, -141.9465) -> (-41.5019, -134.0964)
  arc A33 (-38.7691, -131.314) -> (-41.5019, -134.0964) centre (-40.1368, -132.704) ccw
  line L27 (-38.7691, -131.314) -> (-31.2739, -131.314)
  arc A34 (-28.4537, -134.0071) -> (-31.2739, -131.314) centre (-29.8857, -132.6834) ccw
  line L28 (-68.4537, -114.0071) -> (-68.4537, -121.9513)
  arc A35 (-71.1924, -124.7264) -> (-68.4537, -121.9513) centre (-69.79, -123.3716) ccw
  line L29 (-71.1924, -124.7264) -> (-78.7712, -124.7264)
  arc A36 (-81.5019, -121.9465) -> (-78.7712, -124.7264) centre (-80.0802, -123.2811) ccw
  line L30 (-81.5019, -121.9465) -> (-81.5019, -114.0964)
  arc A37 (-78.7691, -111.314) -> (-81.5019, -114.0964) centre (-80.1368, -112.704) ccw
  line L31 (-78.7691, -111.314) -> (-71.2739, -111.314)
  arc A38 (-68.4537, -114.0071) -> (-71.2739, -111.314) centre (-69.8857, -112.6834) ccw
  line L32 (-68.4537, -134.0071) -> (-68.4537, -141.9513)
  arc A39 (-71.1924, -144.7264) -> (-68.4537, -141.9513) centre (-69.79, -143.3716) ccw
  line L33 (-71.1924, -144.7264) -> (-78.7712, -144.7264)
  arc A40 (-81.5019, -141.9465) -> (-78.7712, -144.7264) centre (-80.0802, -143.2811) ccw
  line L34 (-81.5019, -141.9465) -> (-81.5019, -134.0964)
  arc A41 (-78.7691, -131.314) -> (-81.5019, -134.0964) centre (-80.1368, -132.704) ccw
  line L35 (-78.7691, -131.314) -> (-71.2739, -131.314)
  arc A42 (-68.4537, -134.0071) -> (-71.2739, -131.314) centre (-69.8857, -132.6834) ccw
  line L36 (-8.4537, -114.0071) -> (-8.4537, -121.9513)
  arc A43 (-11.1924, -124.7264) -> (-8.4537, -121.9513) centre (-9.79, -123.3716) ccw
  line L37 (-11.1924, -124.7264) -> (-18.7712, -124.7264)
  arc A44 (-21.5019, -121.9465) -> (-18.7712, -124.7264) centre (-20.0802, -123.2811) ccw
  line L38 (-21.5019, -121.9465) -> (-21.5019, -114.0964)
  arc A45 (-18.7691, -111.314) -> (-21.5019, -114.0964) centre (-20.1368, -112.704) ccw
  line L39 (-18.7691, -111.314) -> (-11.2739, -111.314)
  arc A46 (-8.4537, -114.0071) -> (-11.2739, -111.314) centre (-9.8857, -112.6834) ccw
  line L40 (-68.4537, -94.0071) -> (-68.4537, -101.9513)
  arc A47 (-71.1924, -104.7264) -> (-68.4537, -101.9513) centre (-69.79, -103.3716) ccw
  line L41 (-71.1924, -104.7264) -> (-78.7712, -104.7264)
  arc A48 (-81.5019, -101.9465) -> (-78.7712, -104.7264) centre (-80.0802, -103.2811) ccw
  line L42 (-81.5019, -101.9465) -> (-81.5019, -94.0964)
  arc A49 (-78.7691, -91.314) -> (-81.5019, -94.0964) centre (-80.1368, -92.704) ccw
  line L43 (-78.7691, -91.314) -> (-71.2739, -91.314)
  arc A50 (-68.4537, -94.0071) -> (-71.2739, -91.314) centre (-69.8857, -92.6834) ccw
  circle A51 centre (-116, -92.5) radius 3.275
  line L44 (-68.4537, -154.0071) -> (-68.4537, -161.9513)
  arc A52 (-71.1924, -164.7264) -> (-68.4537, -161.9513) centre (-69.79, -163.3716) ccw
  line L45 (-71.1924, -164.7264) -> (-78.7712, -164.7264)
  arc A53 (-81.5019, -161.9465) -> (-78.7712, -164.7264) centre (-80.0802, -163.2811) ccw
  line L46 (-81.5019, -161.9465) -> (-81.5019, -154.0964)
  arc A54 (-78.7691, -151.314) -> (-81.5019, -154.0964) centre (-80.1368, -152.704) ccw
  line L47 (-78.7691, -151.314) -> (-71.2739, -151.314)
  arc A55 (-68.4537, -154.0071) -> (-71.2739, -151.314) centre (-69.8857, -152.6834) ccw
  circle A56 centre (-133, -143.5) radius 3.275
  line L48 (-48.4537, -74.0071) -> (-48.4537, -81.9513)
  arc A57 (-51.1924, -84.7264) -> (-48.4537, -81.9513) centre (-49.79, -83.3716) ccw
  line L49 (-51.1924, -84.7264) -> (-58.7712, -84.7264)
  arc A58 (-61.5019, -81.9465) -> (-58.7712, -84.7264) centre (-60.0802, -83.2811) ccw
  line L50 (-61.5019, -81.9465) -> (-61.5019, -74.0964)
  arc A59 (-58.7691, -71.314) -> (-61.5019, -74.0964) centre (-60.1368, -72.704) ccw
  line L51 (-58.7691, -71.314) -> (-51.2739, -71.314)
  arc A60 (-48.4537, -74.0071) -> (-51.2739, -71.314) centre (-49.8857, -72.6834) ccw
  circle A61 centre (-133, -126.5) radius 3.275
  circle A62 centre (-99, -92.5) radius 3.275
  line L52 (-48.4537, -94.0071) -> (-48.4537, -101.9513)
  arc A63 (-51.1924, -104.7264) -> (-48.4537, -101.9513) centre (-49.79, -103.3716) ccw
  line L53 (-51.1924, -104.7264) -> (-58.7712, -104.7264)
  arc A64 (-61.5019, -101.9465) -> (-58.7712, -104.7264) centre (-60.0802, -103.2811) ccw
  line L54 (-61.5019, -101.9465) -> (-61.5019, -94.0964)
  arc A65 (-58.7691, -91.314) -> (-61.5019, -94.0964) centre (-60.1368, -92.704) ccw
  line L55 (-58.7691, -91.314) -> (-51.2739, -91.314)
  arc A66 (-48.4537, -94.0071) -> (-51.2739, -91.314) centre (-49.8857, -92.6834) ccw
  line L56 (-8.4537, -134.0071) -> (-8.4537, -141.9513)
  arc A67 (-11.1924, -144.7264) -> (-8.4537, -141.9513) centre (-9.79, -143.3716) ccw
  line L57 (-11.1924, -144.7264) -> (-18.7712, -144.7264)
  arc A68 (-21.5019, -141.9465) -> (-18.7712, -144.7264) centre (-20.0802, -143.2811) ccw
  line L58 (-21.5019, -141.9465) -> (-21.5019, -134.0964)
  arc A69 (-18.7691, -131.314) -> (-21.5019, -134.0964) centre (-20.1368, -132.704) ccw
  line L59 (-18.7691, -131.314) -> (-11.2739, -131.314)
  arc A70 (-8.4537, -134.0071) -> (-11.2739, -131.314) centre (-9.8857, -132.6834) ccw
  circle A71 centre (-116, -143.5) radius 3.275
  line L60 (-8.4537, -154.0071) -> (-8.4537, -161.9513)
  arc A72 (-11.1924, -164.7264) -> (-8.4537, -161.9513) centre (-9.79, -163.3716) ccw
  line L61 (-11.1924, -164.7264) -> (-18.7712, -164.7264)
  arc A73 (-21.5019, -161.9465) -> (-18.7712, -164.7264) centre (-20.0802, -163.2811) ccw
  line L62 (-21.5019, -161.9465) -> (-21.5019, -154.0964)
  arc A74 (-18.7691, -151.314) -> (-21.5019, -154.0964) centre (-20.1368, -152.704) ccw
  line L63 (-18.7691, -151.314) -> (-11.2739, -151.314)
  arc A75 (-8.4537, -154.0071) -> (-11.2739, -151.314) centre (-9.8857, -152.6834) ccw
  line L64 (-48.4537, -114.0071) -> (-48.4537, -121.9513)
  arc A76 (-51.1924, -124.7264) -> (-48.4537, -121.9513) centre (-49.79, -123.3716) ccw
  line L65 (-51.1924, -124.7264) -> (-58.7712, -124.7264)
  arc A77 (-61.5019, -121.9465) -> (-58.7712, -124.7264) centre (-60.0802, -123.2811) ccw
  line L66 (-61.5019, -121.9465) -> (-61.5019, -114.0964)
  arc A78 (-58.7691, -111.314) -> (-61.5019, -114.0964) centre (-60.1368, -112.704) ccw
  line L67 (-58.7691, -111.314) -> (-51.2739, -111.314)
  arc A79 (-48.4537, -114.0071) -> (-51.2739, -111.314) centre (-49.8857, -112.6834) ccw
  circle A80 centre (-133, -160.5) radius 3.275
  line L68 (-48.4537, -154.0071) -> (-48.4537, -161.9513)
  arc A81 (-51.1924, -164.7264) -> (-48.4537, -161.9513) centre (-49.79, -163.3716) ccw
  line L69 (-51.1924, -164.7264) -> (-58.7712, -164.7264)
  arc A82 (-61.5019, -161.9465) -> (-58.7712, -164.7264) centre (-60.0802, -163.2811) ccw
  line L70 (-61.5019, -161.9465) -> (-61.5019, -154.0964)
  arc A83 (-58.7691, -151.314) -> (-61.5019, -154.0964) centre (-60.1368, -152.704) ccw
  line L71 (-58.7691, -151.314) -> (-51.2739, -151.314)
  arc A84 (-48.4537, -154.0071) -> (-51.2739, -151.314) centre (-49.8857, -152.6834) ccw
  line L72 (-28.4537, -114.0071) -> (-28.4537, -121.9513)
  arc A85 (-31.1924, -124.7264) -> (-28.4537, -121.9513) centre (-29.79, -123.3716) ccw
  line L73 (-31.1924, -124.7264) -> (-38.7712, -124.7264)
  arc A86 (-41.5019, -121.9465) -> (-38.7712, -124.7264) centre (-40.0802, -123.2811) ccw
  line L74 (-41.5019, -121.9465) -> (-41.5019, -114.0964)
  arc A87 (-38.7691, -111.314) -> (-41.5019, -114.0964) centre (-40.1368, -112.704) ccw
  line L75 (-38.7691, -111.314) -> (-31.2739, -111.314)
  arc A88 (-28.4537, -114.0071) -> (-31.2739, -111.314) centre (-29.8857, -112.6834) ccw
  circle A89 centre (-99, -160.5) radius 3.275
  circle A90 centre (-99, -126.5) radius 3.275
  circle A91 centre (-116, -109.5) radius 3.275
  line L76 (-28.4537, -94.0071) -> (-28.4537, -101.9513)
  arc A92 (-31.1924, -104.7264) -> (-28.4537, -101.9513) centre (-29.79, -103.3716) ccw
  line L77 (-31.1924, -104.7264) -> (-38.7712, -104.7264)
  arc A93 (-41.5019, -101.9465) -> (-38.7712, -104.7264) centre (-40.0802, -103.2811) ccw
  line L78 (-41.5019, -101.9465) -> (-41.5019, -94.0964)
  arc A94 (-38.7691, -91.314) -> (-41.5019, -94.0964) centre (-40.1368, -92.704) ccw
  line L79 (-38.7691, -91.314) -> (-31.2739, -91.314)
  arc A95 (-28.4537, -94.0071) -> (-31.2739, -91.314) centre (-29.8857, -92.6834) ccw
  line L80 (-28.4537, -154.0071) -> (-28.4537, -161.9513)
  arc A96 (-31.1924, -164.7264) -> (-28.4537, -161.9513) centre (-29.79, -163.3716) ccw
  line L81 (-31.1924, -164.7264) -> (-38.7712, -164.7264)
  arc A97 (-41.5019, -161.9465) -> (-38.7712, -164.7264) centre (-40.0802, -163.2811) ccw
  line L82 (-41.5019, -161.9465) -> (-41.5019, -154.0964)
  arc A98 (-38.7691, -151.314) -> (-41.5019, -154.0964) centre (-40.1368, -152.704) ccw
  line L83 (-38.7691, -151.314) -> (-31.2739, -151.314)
  arc A99 (-28.4537, -154.0071) -> (-31.2739, -151.314) centre (-29.8857, -152.6834) ccw
  circle A100 centre (-133, -109.5) radius 3.275
  line L84 (-68.4537, -74.0071) -> (-68.4537, -81.9513)
  arc A101 (-71.1924, -84.7264) -> (-68.4537, -81.9513) centre (-69.79, -83.3716) ccw
  line L85 (-71.1924, -84.7264) -> (-78.7712, -84.7264)
  arc A102 (-81.5019, -81.9465) -> (-78.7712, -84.7264) centre (-80.0802, -83.2811) ccw
  line L86 (-81.5019, -81.9465) -> (-81.5019, -74.0964)
  arc A103 (-78.7691, -71.314) -> (-81.5019, -74.0964) centre (-80.1368, -72.704) ccw
  line L87 (-78.7691, -71.314) -> (-71.2739, -71.314)
  arc A104 (-68.4537, -74.0071) -> (-71.2739, -71.314) centre (-69.8857, -72.6834) ccw
  line L88 (-75.1019, -28.3976) -> (-80.9582, -31.7787)
  arc A105 (-83.1621, -31.7787) -> (-80.9582, -31.7787) centre (-82.0601, -29.87) ccw
  line L89 (-83.1621, -31.7787) -> (-87.1295, -29.4881)
  arc A106 (-87.1295, -28.5338) -> (-87.1295, -29.4881) centre (-86.854, -29.0109) ccw
  line L90 (-87.1295, -28.5338) -> (-75.1019, -21.5897)
  arc A107 (-72.8981, -21.5897) -> (-75.1019, -21.5897) centre (-74, -23.4983) ccw
  line L91 (-72.8981, -21.5897) -> (-61.146, -28.3747)
  arc A108 (-60.0441, -30.2834) -> (-61.146, -28.3747) centre (-62.248, -30.2834) ccw
  line L92 (-60.0441, -30.2834) -> (-60.0441, -43.8607)
  arc A109 (-61.0054, -45.6809) -> (-60.0441, -43.8607) centre (-62.248, -43.8607) ccw
  line L93 (-61.0054, -45.6809) -> (-72.8981, -52.5471)
  arc A110 (-75.1019, -52.5471) -> (-72.8981, -52.5471) centre (-74, -50.6385) ccw
  line L94 (-75.1019, -52.5471) -> (-87.1295, -45.603)
  arc A111 (-87.1295, -44.6487) -> (-87.1295, -45.603) centre (-86.854, -45.1259) ccw
  line L95 (-87.1295, -44.6487) -> (-83.1621, -42.3581)
  arc A112 (-80.9582, -42.3581) -> (-83.1621, -42.3581) centre (-82.0601, -44.2667) ccw
  line L96 (-80.9582, -42.3581) -> (-75.1019, -45.7392)
  arc A113 (-75.1019, -45.7392) -> (-72.8981, -45.7392) centre (-74, -43.8306) ccw
  line L97 (-72.8981, -45.7392) -> (-67.0418, -42.3581)
  arc A114 (-67.0418, -42.3581) -> (-65.9399, -40.4495) centre (-68.1438, -40.4495) ccw
  line L98 (-65.9399, -40.4495) -> (-65.9399, -33.6873)
  arc A115 (-65.9399, -33.6873) -> (-67.0418, -31.7787) centre (-68.1438, -33.6873) ccw
  line L99 (-67.0418, -31.7787) -> (-72.8981, -28.3976)
  arc A116 (-72.8981, -28.3976) -> (-75.1019, -28.3976) centre (-74, -30.3062) ccw
  arc A117 (-72.8983, -14.2882) -> (-75.1022, -14.2882) centre (-74.0002, -16.1968) ccw
  line L100 (-75.1022, -14.2882) -> (-93.1774, -24.7242)
  arc A118 (-93.1774, -24.7242) -> (-94.2793, -26.6328) centre (-92.0754, -26.6328) ccw
  line L101 (-94.2793, -26.6328) -> (-94.2791, -47.5044)
  arc A119 (-94.2791, -47.5044) -> (-93.1771, -49.413) centre (-92.0752, -47.5044) ccw
  line L102 (-93.1771, -49.413) -> (-75.1017, -59.8486)
  arc A120 (-75.1017, -59.8486) -> (-72.8978, -59.8486) centre (-73.9998, -57.94) ccw
  line L103 (-72.8978, -59.8486) -> (-54.8226, -49.4126)
  arc A121 (-54.8226, -49.4126) -> (-53.7207, -47.504) centre (-55.9246, -47.504) ccw
  line L104 (-53.7207, -47.504) -> (-53.7209, -26.6324)
  arc A122 (-53.7209, -26.6324) -> (-54.8229, -24.7238) centre (-55.9248, -26.6324) ccw
  line L105 (-54.8229, -24.7238) -> (-72.8983, -14.2882)
equation "d6 = PocketWidth"
equation "d14 = d13"
equation "d15 = d13"
equation "d16 = d13"
equation "d28 = ToolPocketDiameter"
equation "d49 = d51"
equation "d50 = d51"
equation "PocketWidth = 13 mm"
equation "ToolPocketDiameter = 6.55 mm"
